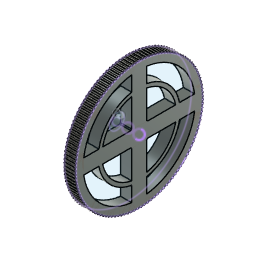
Robo Wheel v3 (Autodesk Fusion 360 design; units mm, degrees)
Autodesk Fusion 360 part; units mm, degrees
sketch "Sketch1" plane through (0, 0, 0) normal (1, 0, 0) x (0, 1, 0)
  circle A0 centre (0, 0) radius 85
  circle A1 centre (0, 0) radius 75
  circle A2 centre (0, 0) radius 15
  arc A3 (-10, 48.9898) -> (-48.9898, 10) centre (0, 0) ccw
  arc A4 (-10, 54.0833) -> (-54.0833, 10) centre (0, 0) ccw
  arc A5 (-48.9898, -10) -> (-10, -48.9898) centre (0, 0) ccw
  arc A6 (-54.0833, -10) -> (-10, -54.0833) centre (0, 0) ccw
  arc A7 (10.0447, -48.9806) -> (48.9898, -10) centre (0, 0) ccw
  arc A8 (48.9898, 10) -> (10.0447, 48.9806) centre (0, 0) ccw
  arc A9 (10.0447, -54.075) -> (54.0833, -10) centre (0, 0) ccw
  arc A10 (54.0833, 10) -> (10.0447, 54.075) centre (0, 0) ccw
  line L0 (-74.3303, 10) -> (-54.0833, 10)
  line L1 (-48.9898, 10) -> (-11.1803, 10)
  line L2 (-74.3303, -10) -> (-54.0833, -10)
  line L3 (-48.9898, -10) -> (-11.1803, -10)
  line L4 (-10, 11.1803) -> (-10, 48.9898)
  line L5 (-10, 54.0833) -> (-10, 74.3303)
  line L6 (10.0447, 74.3243) -> (10.0447, 54.075)
  line L7 (10.0447, 48.9806) -> (10.0447, 11.1402)
  line L8 (11.1803, 10) -> (48.9898, 10)
  line L9 (54.0833, 10) -> (74.3303, 10)
  line L10 (11.1803, -10) -> (48.9898, -10)
  line L11 (54.0833, -10) -> (74.3303, -10)
  line L12 (10.0447, -11.1402) -> (10.0447, -48.9806)
  line L13 (10.0447, -54.075) -> (10.0447, -74.3243)
  line L14 (-10, -11.1803) -> (-10, -48.9898)
  line L15 (-10, -54.0833) -> (-10, -74.3303)
  dimension "d1" = 170
  dimension "d2" = 150
  constraint coincident A0.centre A1.centre
  constraint concentric A1 A2
  constraint coincident A2 L4.start
  constraint coincident A1 L5.end
  constraint coincident A1 L6.start
  constraint coincident A2 L7.end
  constraint coincident A1 L0.start
  constraint coincident A2 L1.end
  constraint coincident A1 L2.start
  constraint coincident A2 L3.end
  constraint coincident A2 L14.start
  constraint coincident A1 L15.end
  constraint coincident A2 L12.start
  constraint coincident A1 L13.end
  constraint coincident A2 L8.start
  constraint coincident A1 L9.end
  constraint coincident A2 L10.start
  constraint coincident A1 L11.end
  constraint concentric A1 A3
  constraint concentric A1 A4
  constraint concentric A3 A5
  constraint concentric A4 A6
  constraint concentric A5 A7
  constraint concentric A6 A9
  constraint concentric A7 A8
  constraint concentric A9 A10
  constraint collinear L0 L1
  constraint collinear L2 L3
  constraint collinear L4 L5
  constraint collinear L6 L7
  constraint collinear L8 L9
  constraint collinear L10 L11
  constraint collinear L12 L13
  constraint collinear L14 L15
  measures "d1" diameter of A0
  measures "d2" diameter of A1
extrude "Extrude1" add sketch "Sketch1" along normal blind 15 contours A0 | A1 A4 A6 A9 A10 L0 L2 L5 L6 L9 L11 L13 L15 | A2
sketch "Sketch2" plane through (0, 0, 0) normal (0, 1, 0) x (1, 0, 0)
  circle A0 through (15, -85, 0) (15, 42.5, 73.6122) (15, 42.5, -73.6122)
  circle A1 through (0, -85, 0) (0, 42.5, 73.6122) (0, 42.5, -73.6122)
sketch "Sketch3" plane through (0, 0, 0) normal (1, 0, 0) x (0, 1, 0)
  circle A0 through (85, 0, 15) (-42.5, 73.6122, 15) (-42.5, -73.6122, 15)
  circle A1 centre (0, 0) radius 85
  arc A2 (45.0898, 72.0549) -> (43.382, 73.0958) centre (44.239, 72.5804) ccw
  dimension "d7" = 2
  constraint coincident A1 A2.centre
  constraint coincident A1 A2.end
  constraint coincident A1 A2.start
  measures "d7" diameter of A2
extrude "Extrude2" add sketch "Sketch3" along normal blind 15 contours A1 A2
pattern_circular "C-Pattern1" count 120 over 360 about axis through (0, 0, 0) along (1, 0, 0) of "Extrude2"
sketch "Sketch4" plane through (0, 0, 0) normal (1, 0, 0) x (0, 1, 0)
sketch "Sketch5" plane through (0, 0, 0) normal (0, 1, 0) x (1, 0, 0)
sketch "Sketch6" plane through (0, 0, 0) normal (1, 0, 0) x (0, 1, 0)
  circle A0 centre (0, 0) radius 1.75
  circle A1 centre (0, 0) radius 10
  dimension "d12" = 3.5
  constraint coincident A0.centre A1.centre
  measures "d12" diameter of A0
extrude "Extrude3" add sketch "Sketch6" against normal blind 15
sketch "Sketch7" plane through (0, 0, 0) normal (1, 0, 0) x (0, 1, 0)
  circle A0 through (10, 0, -15) (-5, 8.6603, -15) (-5, -8.6603, -15)
  line L0 (-0.1321, 9.9991, -15) -> (-0.1321, 9.9991, -10)
  dimension "d15" = 5
hole "Hole1" at (-8.7014, 0, 10) direction (0, 0, -1) diameter 3 depth 9.5 tip angle 180
sketch "Sketch8" plane through (0, 0, 0) normal (1, 0, 0) x (0, 1, 0)
  circle A0 centre (0, 0) radius 3.5
  constraint coincident A0.centre origin
extrude "Extrude4" cut sketch "Sketch8" against normal blind 15
